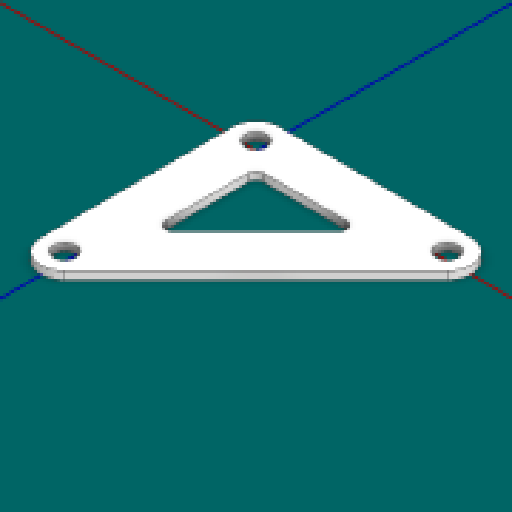
# Autodesk Inventor part: right_angle_gusset
Saved by Autodesk Inventor 2025 (Build 290162000, 162)
## iProperties
Created: 2024-08-17
Part Number: right_angle_gusset
Material: Acetal Resin, White
Document SubType Name: Modeling
Designer: averey
Density: 1.425 g/cm^3
Appearance: Smooth - White
d0: 0.375 in
d1: 0.375 in
d2: 0.375 in
d5: 0.375 in
d6: 0.063 in
d7: 0.063 in
Author: averey
Autodesk Inventor part; units mm, degrees
ref_plane "YZ Plane" through (0, 0, 0) normal (1, 0, 0) x (0, 1, 0)
ref_plane "XZ Plane" through (0, 0, 0) normal (0, 1, 0) x (-1, 0, 0)
ref_plane "XY Plane" through (0, 0, 0) normal (0, 0, 1) x (1, 0, 0)
sketch "main" plane through (0, 0, 0) normal (0, 0, 1) x (1, 0, 0)
  circle A0 centre (19.7324, 21.1672) radius 2.1844
  circle A1 centre (19.7324, -16.9328) radius 2.1844
  circle A2 centre (-18.3676, -16.9328) radius 2.1844
  arc A3 (24.4949, 21.1672) -> (16.3648, 24.5348) centre (19.7324, 21.1672) ccw
  arc A4 (-21.7352, -13.5652) -> (-18.3676, -21.6953) centre (-18.3676, -16.9328) ccw
  arc A5 (19.7324, -21.6953) -> (24.4949, -16.9317) centre (19.7324, -16.9328) ccw
  line L0 (19.7324, -21.6953) -> (-18.3676, -21.6953)
  line L1 (24.4949, 21.1672) -> (24.4949, -16.9317)
  line L2 (16.3648, 24.5348) -> (-21.7352, -13.5652)
  line L3 (13.3824, -12.1703) -> (-3.0373, -12.1703)
  line L4 (-4.1599, -9.4602) -> (12.2599, 6.9595)
  line L5 (14.9699, 5.837) -> (14.9699, -10.5828)
  arc A6 (13.3824, -12.1703) -> (14.9699, -10.5828) centre (13.3824, -10.5828) ccw
  arc A7 (14.9699, 5.837) -> (12.2599, 6.9595) centre (13.3824, 5.837) ccw
  arc A8 (-4.1599, -9.4602) -> (-3.0373, -12.1703) centre (-3.0373, -10.5828) ccw
  point P0 (6.6792, -3.8964)
  dimension "d0" = 9.525
  dimension "d1" = 9.525
  dimension "d2" = 9.525
  dimension "d5" = 9.525
  dimension "d6" = 1.5875
  dimension "d7" = 1.5875
  measures "d0" diameter of A3
  measures "d1" diameter of A4
  measures "d2" diameter of A5
  measures "d5" distance between parallel lines of L1 L5
  measures "d6" radius of A6
  measures "d7" radius of A7
sketch "Sketch1" plane through (0, 0, 0) normal (0, 1, 0) x (-1, 0, 0)
  circle A0 centre (0, 38.1) radius 2.1844
  circle A1 centre (0, 0) radius 2.1844
  circle A2 centre (-38.1, 0) radius 2.1844
  arc A3 (4.7625, 38.1) -> (-3.3676, 41.4676) centre (0, 38.1) ccw
  arc A4 (-41.4676, 3.3676) -> (-38.1, -4.7625) centre (-38.1, 0) ccw
  arc A5 (0, -4.7625) -> (4.7625, 0.0011) centre (0, 0) ccw
  line L0 (0, -4.7625) -> (-38.1, -4.7625)
  line L1 (4.7625, 38.1) -> (4.7625, 0.0011)
  line L2 (-3.3676, 41.4676) -> (-41.4676, 3.3676)
  line L3 (-6.35, 4.7625) -> (-22.7697, 4.7625)
  line L4 (-23.8923, 7.4725) -> (-7.4725, 23.8923)
  line L5 (-4.7625, 22.7697) -> (-4.7625, 6.35)
  arc A6 (-6.35, 4.7625) -> (-4.7625, 6.35) centre (-6.35, 6.35) ccw
  arc A7 (-4.7625, 22.7697) -> (-7.4725, 23.8923) centre (-6.35, 22.7697) ccw
  arc A8 (-23.8923, 7.4725) -> (-22.7697, 4.7625) centre (-22.7697, 6.35) ccw
  constraints: 1 other
extrude "Extrusion1" add sketch "Sketch1" along normal blind 1.5875
body "Solid1"
